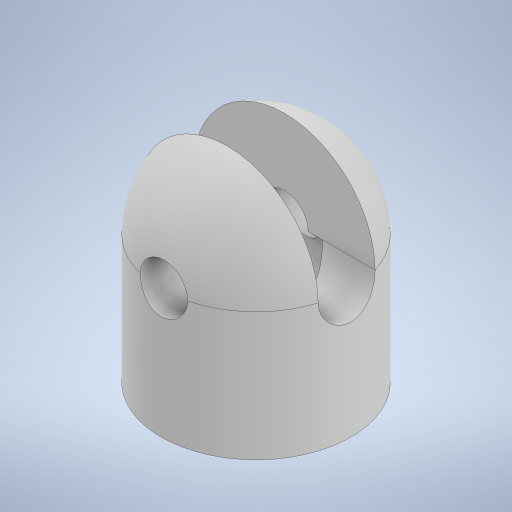
# Autodesk Inventor part: cupula_obj5
Saved by Autodesk Inventor 2023.2 (Build 272271030, 271C)
## iProperties
Created: 2023-02-25
Part Number: cupula_obj5
Material: Generic
Document SubType Name: Modeling
Designer: Cris Pat
Density: 1 g/cm^3
Appearance: Default
Author: Cris Pat
Autodesk Inventor part; units mm, degrees
ref_plane "YZ Plane" through (0, 0, 0) normal (1, 0, 0) x (0, 1, 0)
ref_plane "XZ Plane" through (0, 0, 0) normal (0, 1, 0) x (-1, 0, 0)
ref_plane "XY Plane" through (0, 0, 0) normal (0, 0, 1) x (1, 0, 0)
sketch "Sketch1" plane through (0, 0, 0) normal (0, 1, 0) x (-1, 0, 0)
  circle A0 centre (0, 0) radius 20
  dimension "d0" = 40
  constraints: 1 centre point, 1 coincident
  measures "d0" diameter of A0
extrude "Extrusion1" add sketch "Sketch1" along normal blind 27
sketch "Sketch2" plane through (0, 27, 0) normal (0, 1, 0) x (1, 0, 0)
  circle A0 centre (0, 0) radius 20 construction
  circle A1 centre (0, 0) radius 20 construction
  line L0 (0, -20) -> (0, 20) construction
  arc A2 (0, -20) -> (0, 20) centre (0, 0) ccw
  line L1 (0, -20) -> (0, 20)
  dimension "d3" = 40
  constraints: 4 end point, 4 point on circle, 1 centre point, 1 collinear, 1 concentric, 1 vertical
  measures "d3" distance of L0.start L0.end
revolve "Revolution1" add sketch "Sketch2" angle 180 about axis through (0, 27, 20) along (0, 0, 1)
sketch "Sketch3" plane through (0, 0, 0) normal (0, 0, 1) x (1, 0, 0)
  line L0 (20, 27) -> (-20, 27) construction
  line L1 (20, 27) -> (-20, 27) construction
  line L2 (20, 0) -> (-20, 0) construction
  circle A0 centre (0, 27) radius 5
  arc A1 (20, 27) -> (-20, 27) centre (0, 27) ccw construction
  point P0 (0, 0)
  point P1 (0, 0)
  dimension "d5" = 10
  constraints: 2 midpoint, 1 centre point, 1 coincident, 1 vertical alignment
  measures "d5" diameter of A0
extrude "Extrusion2" cut sketch "Sketch3" along normal through all both and the other way through all
sketch "Sketch4" plane through (0, 0, 0) normal (1, 0, 0) x (0, 1, 0)
  line L0 (27, 19.3649) -> (27, 19.3649) construction
  line L1 (27, 19.3649) -> (27, -19.3649) construction
  line L2 (27, -19.3649) -> (27, -19.3649) construction
  line L3 (27, -19.3649) -> (27, 19.3649) construction
  line L4 (27, 19.3649) -> (27, 19.3649) construction
  line L5 (27, -19.3649) -> (27, -19.3649) construction
  line L6 (0, -20) -> (0, 20) construction
  line L7 (27, -19.3649) -> (27, 19.3649) construction
  line L8 (27, 19.3649) -> (27, -19.3649) construction
  line L9 (27, -19.3649) -> (27, 19.3649) construction
  arc A0 (27, 6) -> (27, -6) centre (27, 0) ccw
  line L10 (27, -6) -> (47.2684, -6)
  line L11 (27, 6) -> (47.2684, 6)
  line L12 (47.2684, -6) -> (47.2684, 6)
  point P0 (0, 0)
  dimension "d8" = 12
  dimension "d9" = 20.2684
  constraints: 6 end point, 2 horizontal, 2 point on circle, 1 centre point, 1 midpoint, 1 tangent, 1 vertical, 4 other
  measures "d8" diameter of A0
  measures "d9" distance from line of point (27, 0) L12
extrude "Extrusion3" cut sketch "Sketch4" along normal through all both and the other way through all
sketch "Sketch5" plane through (0, 0, 0) normal (0, -1, 0) x (1, 0, 0)
  circle A0 centre (0, 0) radius 10
  dimension "d12" = 20
  constraints: 1 centre point, 1 coincident
  measures "d12" diameter of A0
extrude "Extrusion4" cut sketch "Sketch5" against normal up to surface (27 mm away)
body "Solid1"
